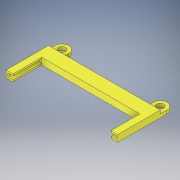
# Autodesk Inventor part: Electronics-Wedge
Saved by Autodesk Inventor 2018 (Build 220112000, 112)
## iProperties
Created: 2018-07-29
Part Number: Electronics-Wedge
Material: Generic
Document SubType Name: Modeling
Designer: jklei
Density: 1 g/cm^3
Appearance: Default
Author: jklei
Autodesk Inventor part; units mm, degrees
ref_plane "YZ Plane" through (0, 0, 0) normal (1, 0, 0) x (0, 1, 0)
ref_plane "XZ Plane" through (0, 0, 0) normal (0, 1, 0) x (-1, 0, 0)
sketch "Sketch1" plane through (0, 0, 0) normal (0, 0, 1) x (1, 0, 0)
  line L0 (0, 0) -> (66, 0)
  line L1 (66, 0) -> (66, 4)
  line L2 (66, 4) -> (0, 4)
  line L3 (0, 4) -> (0, 0)
  dimension "d0" = 66
  dimension "d1" = 4
  constraints: 8 end point, 2 parallel, 1 horizontal, 1 perpendicular
  measures "d0" distance of L2.end L1.end
  measures "d1" distance of L1.end L0.end
extrude "Extrusion1" add sketch "Sketch1" along normal blind 20
sketch "Sketch2" plane through (0, 4, 0) normal (0, 1, 0) x (1, 0, 0)
  line L0 (0, -20) -> (66, -20) projected
  line L1 (4, -20) -> (62, -20)
  line L2 (62, -20) -> (62, -3)
  line L3 (62, -3) -> (4, -3)
  line L4 (4, -3) -> (4, -20)
  line L5 (0, 0) -> (0, -20) projected
  dimension "d4" = 58
  dimension "d5" = 17
  dimension "d6" = 4
  constraints: 8 end point, 2 parallel, 1 horizontal, 1 perpendicular, 1 point on line
  measures "d4" distance of L3.end L2.end
  measures "d5" distance of L2.end L1.end
  measures "d6" distance between parallel lines of L5 L4
extrude "Extrusion2" cut sketch "Sketch2" against normal blind 20
ref_plane "Work Plane1" through (0, 0, 20) normal (0, 0, 1) x (1, 0, 0)
sketch "Sketch3" plane through (0, 0, 20) normal (0, 0, 1) x (1, 0, 0)
  line L0 (4, 0) -> (4, 4) projected
  line L1 (4, 4) -> (0, 4) projected
  line L2 (0, 4) -> (0, 0) projected
  line L3 (0, 0) -> (4, 0) projected
  line L4 (62, 4) -> (62, 0) projected
  line L5 (62, 0) -> (66, 0) projected
  line L6 (66, 0) -> (66, 4) projected
  line L7 (66, 4) -> (62, 4) projected
  line L8 (4, 0) -> (1, 0)
  line L9 (4, 1) -> (4, 0)
  line L10 (1, 3) -> (4, 3)
  line L11 (4, 3) -> (4, 1)
  line L12 (4, 1) -> (1, 1)
  line L13 (1, 1) -> (1, 3)
  line L14 (62, 3) -> (65, 3)
  line L15 (65, 3) -> (65, 1)
  line L16 (65, 1) -> (62, 1)
  line L17 (62, 1) -> (62, 3)
  dimension "d30" = 3
  dimension "d31" = 2
  dimension "d32" = 1
  dimension "d33" = 4
  dimension "d34" = 3
  dimension "d35" = 2
  dimension "d36" = 1
  dimension "d37" = 4
  constraints: 20 end point, 4 parallel, 3 horizontal, 2 perpendicular
  measures "d30" distance of L11.end L12.end
  measures "d31" distance of L10.end L11.end
  measures "d32" distance between parallel lines of L8 L12
  measures "d33" distance between parallel lines of L2 L11
  measures "d34" distance of L15.end L16.end
  measures "d35" distance of L14.end L15.end
  measures "d36" distance between parallel lines of L5 L16
  measures "d37" distance between parallel lines of L6 L17
extrude "Extrusion3" cut sketch "Sketch3" against normal blind 17 contours L12 L13 L10 L0 | L14 L15 L16 L4
sketch "Sketch4" plane through (0, 4, 0) normal (0, 1, 0) x (1, 0, 0)
  line L0 (0, 0) -> (66, 0)
  line L1 (60, 5) -> (10, 5)
  line L2 (0, 5) -> (0, 0)
  line L3 (60, 5) -> (66, 5)
  line L4 (60, 5) -> (0, 5)
  line L5 (4, -20) -> (4, -3) projected
  line L6 (4, -3) -> (62, -3) projected
  line L7 (62, -3) -> (62, -20) projected
  line L8 (66, -20) -> (62, -20) projected
  line L9 (66, 0) -> (66, -20) projected
  line L10 (66, 0) -> (0, 0) projected
  line L11 (0, 0) -> (0, -20) projected
  line L12 (4, -20) -> (0, -20) projected
  line L13 (66, 0) -> (66, 5)
  point P0 (66.0117, 5)
  constraints: 12 end point, 3 point on line, 2 horizontal, 1 collinear, 1 parallel, 1 perpendicular
extrude "Extrusion5" add sketch "Sketch4" against normal blind 4 contours L2 L4 L1 L3 L13 L0
sketch "Sketch6" plane through (4, 0, 3) normal (0, -1, 0) x (1, 0, 0)
  circle A0 centre (58, -12) radius 2.1
  arc A1 (54, -12) -> (62, -12) centre (58, -12) ccw
  line L0 (54, -12) -> (54, -8)
  arc A2 (-4, -12) -> (4, -12) centre (0, -12) ccw
  circle A3 centre (0, -12) radius 2.1
  line L1 (4, -12) -> (4, -8)
  line L2 (-4, -12) -> (-4, -8)
  line L3 (62, -8) -> (62, 17) projected
  line L4 (62, -8) -> (-4, -8) projected
  line L5 (62, -8) -> (62, 17) projected
  line L6 (62, -8) -> (62, -12)
  line L7 (-4, 17) -> (-4, -8) projected
  dimension "d40" = 4.2
  dimension "d41" = 8
  dimension "d44" = 8
  dimension "d45" = 4.2
  dimension "d53" = 4
  dimension "d54" = 4
  dimension "d55" = 4
  dimension "d56" = 4
  constraints: 8 end point, 5 point on circle, 4 centre point, 2 coincident, 2 tangent, 1 collinear, 1 parallel, 1 vertical
  measures "d40" diameter of A0
  measures "d41" diameter of A1
  measures "d44" diameter of A2
  measures "d45" diameter of A3
  measures "d53" distance from line of L3 A0.centre
  measures "d54" distance from line of L7 A2.centre
  measures "d55" distance from line of L4 A2.centre
  measures "d56" distance from line of L4 A0.centre
extrude "Extrusion6" add sketch "Sketch6" against normal blind 2
body "Solid1"
